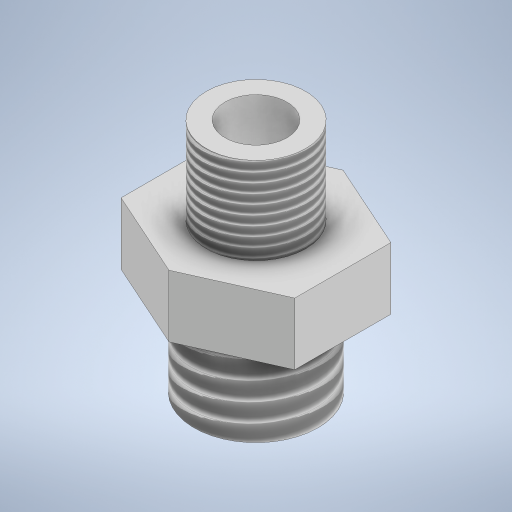
# Autodesk Inventor part: 1-HUDSON-8-29-TDR HAND PUMP BODY TOP OUTLET
Saved by Autodesk Inventor 2024.2 (Build 282272000, 272)
## iProperties
Created: 2024-11-02
Part Number: 1-HUDSON-8-29-TDR HAND PUMP BODY TOP OUTLET
Material: Genérico
Document SubType Name: Modeling
Designer: brene
Density: 1 g/cm^3
Appearance: Valor por defecto
Author: brene
Autodesk Inventor part; units mm, degrees
ref_plane "YZ Plane" through (0, 0, 0) normal (1, 0, 0) x (0, 1, 0)
ref_plane "XZ Plane" through (0, 0, 0) normal (0, 1, 0) x (-1, 0, 0)
ref_plane "XY Plane" through (0, 0, 0) normal (0, 0, 1) x (1, 0, 0)
sketch "Boceto1" plane through (0, 0, 0) normal (0, 0, 1) x (1, 0, 0)
  line L0 (0, 9.3809) -> (0, -9.3809)
  line L1 (-19.2892, 0) -> (19.2892, 0) construction
  line L2 (0, 7) -> (4, 7)
  line L3 (4, 0) -> (4, 7)
  line L4 (4, 0) -> (7, 0)
  line L5 (7, 0) -> (7, -5)
  line L6 (7, -5) -> (0, -5)
  line L7 (5, -5) -> (5, -12)
  line L8 (5, -12) -> (0, -12)
  line L9 (2.5, 7) -> (2.5, 0)
  line L10 (2, -5) -> (2, -10)
  line L11 (2.5, 0) -> (2.5, -0.5101)
  line L12 (2.5, -0.5101) -> (2, -0.5101)
  line L13 (2, -5) -> (2, -0.5101)
  line L14 (2, -10) -> (1, -10)
  line L15 (1, -10) -> (1, -12)
  point P0 (0, 0)
  point P1 (0, 0)
  dimension "d0" = 14
  dimension "d1" = 10
  dimension "d2" = 8
  dimension "d3" = 5
  dimension "d4" = 4
  dimension "d5" = 2
  dimension "d6" = 2
  dimension "d7" = 7
  dimension "d8" = 5
  dimension "d9" = 7
  constraints: 32 end point, 10 point on line, 8 perpendicular, 4 vertical, 3 horizontal, 2 midpoint, 1 coincident
  measures "d0" diameter of L5 L0
  measures "d1" diameter of L7 L0
  measures "d2" diameter of L3 L0
  measures "d3" diameter of L9 L0
  measures "d4" diameter of L13 L0
  measures "d5" distance of L15.end L14.end
  measures "d6" diameter of L15 L0
  measures "d7" distance of L3.start L2.end
  measures "d8" distance of L4.end L5.end
  measures "d9" distance of L7.start L7.end
revolve "Revolución1" add sketch "Boceto1" angle 360 about axis through (0, 9.3809, 0) along (0, -1, 0) contours L2 L3 L4 L5 L6 L13 L12 L11 L9 | L6 L7 L8 L15 L14 L10
sketch "Boceto2" plane through (0, 0, 0) normal (0, 1, 0) x (1, 0, 0)
  circle A0 centre (0, 0) radius 2.5 projected
  circle A1 centre (0, 0) radius 4 projected
  circle A2 centre (0, 0) radius 4 projected
  circle A3 centre (0, 0) radius 7 projected
  line L0 (7, 3.875) -> (7, -3.875)
  line L1 (-7, 3.875) -> (-7, -3.875)
  circle A4 centre (0, 0) radius 7 projected
  line L2 (-7, 3.875) -> (0.0154, 7)
  line L3 (0.0154, 7) -> (7, 3.875)
  line L4 (-7, -3.875) -> (-0.0154, -7)
  line L5 (-0.0154, -7) -> (7, -3.875)
  arc A5 (0.0154, 7) -> (-5.214, 4.6706) centre (0, 0) ccw
  circle A6 centre (0, 0) radius 7 projected
  arc A7 (5.2088, 4.6764) -> (0.0154, 7) centre (0, 0) ccw
  arc A8 (-0.0154, -7) -> (5.214, -4.6706) centre (0, 0) ccw
  arc A9 (-5.2088, -4.6764) -> (-0.0154, -7) centre (0, 0) ccw
  point P0 (0, 0)
  point P1 (7, 0)
  point P2 (-7, 0)
  point P3 (-0.0154, -7)
  point P4 (-0.0154, -7)
  point P5 (-5.2088, -4.6764)
  point P6 (5.214, -4.6706)
  point P7 (5.2088, 4.6764)
  point P8 (-5.214, 4.6706)
  dimension "d15" = 14
  dimension "d27" = 7.75
  dimension "d28" = 14
  dimension "d29" = 14
  dimension "d30" = 7.75
  dimension "d51" = 7
  dimension "d52" = 1.786
  dimension "d53" = 1.7913
  dimension "d54" = 7.0154
  dimension "d55" = 7.0154
  dimension "d56" = 12.7918
  dimension "d57" = 12.2088
  dimension "d58" = 12.7918
  dimension "d59" = 12.214
  dimension "d60" = 4.2619
  dimension "d61" = 7
  dimension "d62" = 7
  dimension "d63" = 7
  constraints: 14 point on circle, 12 end point, 7 point on line, 5 tangent, 4 centre point, 2 midpoint, 2 parallel, 2 vertical, 6 other
  measures "d15" diameter of A3
  measures "d27" distance of L1.start L1.end
  measures "d28" distance of L4.end A4.end
  measures "d29" distance of L1.start L0.start
  measures "d30" distance of L0.start L0.end
  measures "d51" radius of A7
  measures "d52" distance from line of point (5.214, -4.671) L0
  measures "d53" distance from line of point (5.209, 4.676) L0
  measures "d54" distance from line of point (-0.015, -7) L0
  measures "d55" distance from line of point (-0.015, -7) L0
  measures "d56" distance from line of point (-0.015, -7) L3
  measures "d57" distance from line of point (-5.209, -4.676) L0
  measures "d58" distance from line of point (-5.209, -4.676) L3
  measures "d59" distance from line of point (-5.214, 4.671) L0
  measures "d60" distance from line of point (-5.214, 4.671) L3
  measures "d61" distance of A4.centre point (-0.015, -7)
  measures "d62" distance of point (5.214, -4.671) A4.centre
  measures "d63" distance of point (5.209, 4.676) A4.centre
extrude "Extrusión1" cut sketch "Boceto2" against normal through all contours L3 A3 | A3 L5 | L2 A3 | A3 L4
extrude "Extrusión2" add sketch "Boceto2" against normal blind 5 contours L0 L5 A3 | A3 L3 L0 | A3 L1 L2 | L4 L1 A3
thread "Rosca2" size "M10x1.5" class "6g" standard "ANSI Metric M Profile" length 7
thread "Rosca3" size "M8x0.75" class "6g" standard "ANSI Metric M Profile" length 7
equation "\"d30\" = d27"
